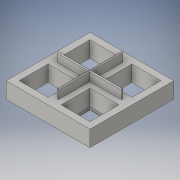
# Autodesk Inventor part: Build Button Top Jig
Saved by Autodesk Inventor 2016 (Build 200138000, 138)
## iProperties
Created: 2017-03-09
Part Number: Build Button Top Jig
Material: Generic
Document SubType Name: Modeling
Designer: Samuel Clay
Density: 1 g/cm^3
Appearance: Default
Author: Samuel Clay
Autodesk Inventor part; units mm, degrees
ref_plane "YZ Plane" through (0, 0, 0) normal (1, 0, 0) x (0, 1, 0)
ref_plane "XZ Plane" through (0, 0, 0) normal (0, 1, 0) x (-1, 0, 0)
ref_plane "XY Plane" through (0, 0, 0) normal (0, 0, 1) x (1, 0, 0)
sketch "Sketch2" plane through (0, 0, 0) normal (0, 1, 0) x (-1, 0, 0)
  line L0 (16.51, -16.51) -> (-16.51, -16.51)
  line L1 (-16.51, -16.51) -> (-16.51, 16.51)
  line L2 (-16.51, 16.51) -> (16.51, 16.51)
  line L3 (16.51, 16.51) -> (16.51, -16.51)
  line L4 (16.51, -16.51) -> (-16.51, 16.51) construction
  line L5 (-16.51, -16.51) -> (16.51, 16.51) construction
  line L6 (13.97, -13.97) -> (-13.97, -13.97)
  line L7 (-13.97, -13.97) -> (-13.97, 13.97)
  line L8 (-13.97, 13.97) -> (13.97, 13.97)
  line L9 (13.97, 13.97) -> (13.97, -13.97)
  line L10 (13.97, -13.97) -> (-13.97, 13.97) construction
  line L11 (-13.97, -13.97) -> (13.97, 13.97) construction
  line L12 (13.97, -2.54) -> (-13.97, -2.54)
  line L13 (-13.97, -2.54) -> (-13.97, 2.54)
  line L14 (-13.97, 2.54) -> (13.97, 2.54)
  line L15 (13.97, 2.54) -> (13.97, -2.54)
  line L16 (13.97, -2.54) -> (-13.97, 2.54) construction
  line L17 (-13.97, -2.54) -> (13.97, 2.54) construction
  line L18 (2.54, -13.97) -> (-2.54, -13.97)
  line L19 (-2.54, -13.97) -> (-2.54, 13.97)
  line L20 (-2.54, 13.97) -> (2.54, 13.97)
  line L21 (2.54, 13.97) -> (2.54, -13.97)
  line L22 (2.54, -13.97) -> (-2.54, 13.97) construction
  line L23 (-2.54, -13.97) -> (2.54, 13.97) construction
  point P0 (0, 0)
  dimension "d20" = 33.02
  dimension "d21" = 33.02
  dimension "d23" = 5.08
  dimension "d24" = 5.08
  dimension "d27" = 13.97
  constraints: 48 end point, 8 midpoint, 8 parallel, 4 horizontal, 4 perpendicular, 3 point on line
  measures "d20" distance of L1.end L2.end
  measures "d21" distance of L0.end L1.end
  measures "d23" distance of L12.end L13.end
  measures "d24" distance of L19.end L20.end
  measures "d27" distance from line of L7 point (0, 0)
extrude "Extrusion3" add sketch "Sketch2" along normal blind 3.175 contours L0 L1 L2 L3 | L6 L19 L12 L21 | L12 L21 L14 L9 | L12 L19 L14 L21 | L12 L7 L14 L19 | L14 L19 L8 L21
sketch "Sketch1" plane through (0, 0, 0) normal (0, 1, 0) x (-1, 0, 0)
  line L0 (19.05, -19.05) -> (-19.05, -19.05)
  line L1 (-19.05, -19.05) -> (-19.05, 19.05)
  line L2 (-19.05, 19.05) -> (19.05, 19.05)
  line L3 (19.05, 19.05) -> (19.05, -19.05)
  line L4 (19.05, -19.05) -> (-19.05, 19.05) construction
  line L5 (-19.05, -19.05) -> (19.05, 19.05) construction
  line L6 (0.254, -12.7) -> (-0.254, -12.7)
  line L7 (-0.254, -12.7) -> (-0.254, 12.7)
  line L8 (-0.254, 12.7) -> (0.254, 12.7)
  line L9 (0.254, 12.7) -> (0.254, -12.7)
  line L10 (0.254, -12.7) -> (-0.254, 12.7) construction
  line L11 (-0.254, -12.7) -> (0.254, 12.7) construction
  line L12 (12.7, -0.254) -> (-12.7, -0.254)
  line L13 (-12.7, -0.254) -> (-12.7, 0.254)
  line L14 (-12.7, 0.254) -> (12.7, 0.254)
  line L15 (12.7, 0.254) -> (12.7, -0.254)
  line L16 (12.7, -0.254) -> (-12.7, 0.254) construction
  line L17 (-12.7, -0.254) -> (12.7, 0.254) construction
  point P0 (0, 0)
  point P1 (0, 0)
  dimension "d0" = 38.1
  dimension "d1" = 38.1
  dimension "d2" = 0.508
  dimension "d3" = 25.4
  dimension "d4" = 0.508
  dimension "d5" = 25.4
  constraints: 36 end point, 8 midpoint, 6 parallel, 3 horizontal, 3 perpendicular
  measures "d0" distance of L1.end L2.end
  measures "d1" distance of L0.end L1.end
  measures "d2" distance of L7.end L8.end
  measures "d3" distance of L13.end L14.end
  measures "d4" distance of L12.end L13.end
  measures "d5" distance between parallel lines of L8 L6
extrude "Extrusion2" add sketch "Sketch1" along normal blind 6.35 contours L6 L7 L12 L9 | L12 L7 L14 L9 | L9 L14 L15 L12 | L12 L13 L14 L7 | L14 L7 L8 L9
sketch "Sketch3" plane through (0, 6.35, 0) normal (0, 1, 0) x (1, 0, 0)
  line L0 (0.254, -0.254) -> (12.7, -0.254) projected
  line L1 (12.7, -0.254) -> (12.7, 0.254) projected
  line L2 (12.7, 0.254) -> (0.254, 0.254) projected
  line L3 (0.254, 0.254) -> (0.254, 12.7) projected
  line L4 (0.254, 12.7) -> (-0.254, 12.7) projected
  line L5 (-0.254, 12.7) -> (-0.254, 0.254) projected
  line L6 (-0.254, 0.254) -> (-12.7, 0.254) projected
  line L7 (-12.7, 0.254) -> (-12.7, -0.254) projected
  line L8 (-12.7, -0.254) -> (-0.254, -0.254) projected
  line L9 (-0.254, -0.254) -> (-0.254, -12.7) projected
  line L10 (-0.254, -12.7) -> (0.254, -12.7) projected
  line L11 (0.254, -12.7) -> (0.254, -0.254) projected
  point P0 (0, 0)
extrude "Extrusion4" add sketch "Sketch3" along normal blind 0.508 draft -25
mirror "Mirror1" about plane through (0, 0, 0) normal (0, 1, 0)
equation "\"d21\" = d20"
body "Solid1"
body "Solid2"
